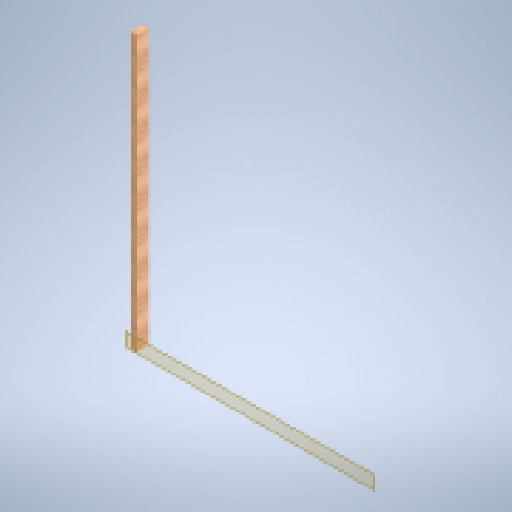
# Autodesk Inventor part: 2X4X92
Saved by Autodesk Inventor 2025 (Build 290162000, 162)
## iProperties
Created: 2024-09-08
Part Number: 2X4X92
Material: Wood (Birch)
Document SubType Name: Modeling
Designer: Win
Density: 0.55 g/cm^3
Appearance: Birch - Natural Polished
Author: Win
Autodesk Inventor part; units mm, degrees
ref_plane "YZ Plane" through (0, 0, 0) normal (1, 0, 0) x (0, 1, 0)
ref_plane "XZ Plane" through (0, 0, 0) normal (0, 1, 0) x (-1, 0, 0)
ref_plane "XY Plane" through (0, 0, 0) normal (0, 0, 1) x (1, 0, 0)
ref_plane "Work Plane1" through (0, 0, 0) normal (0, 0, 1) x (1, 0, 0)
sketch "Sketch1" plane through (0, 0, 0) normal (0, 0, 1) x (1, 0, 0)
  line L0 (965.2, 2336.8) -> (-965.2, 2336.8) projected
  line L1 (-965.2, 2336.8) -> (-965.2, 2235.2) projected
  line L2 (-965.2, 2235.2) -> (965.2, 2235.2) projected
  line L3 (965.2, 2235.2) -> (965.2, 2336.8) projected
  line L4 (-1016, 2286) -> (-965.2, 2286) projected
  line L5 (965.2, 50.8) -> (-965.2, 50.8) projected
  line L6 (-965.2, 50.8) -> (-965.2, -50.8) projected
  line L7 (-965.2, -50.8) -> (965.2, -50.8) projected
  line L8 (965.2, -50.8) -> (965.2, 50.8) projected
  line L9 (-965.2, 2286) -> (-1016, 2286)
  line L10 (-1016, 2286) -> (-1016, -50.8)
  line L11 (-1016, -50.8) -> (-965.2, -50.8)
  line L12 (-965.2, -50.8) -> (-965.2, 2286)
  point P0 (0, 0)
  point P1 (-965.2, 2286)
  constraints: 8 end point, 2 parallel, 1 horizontal, 1 perpendicular
extrude "Extrusion1" add sketch "Sketch1" against normal blind 101.6 contours L1 L12 L6 L11 L10 L4
body "Solid1"
